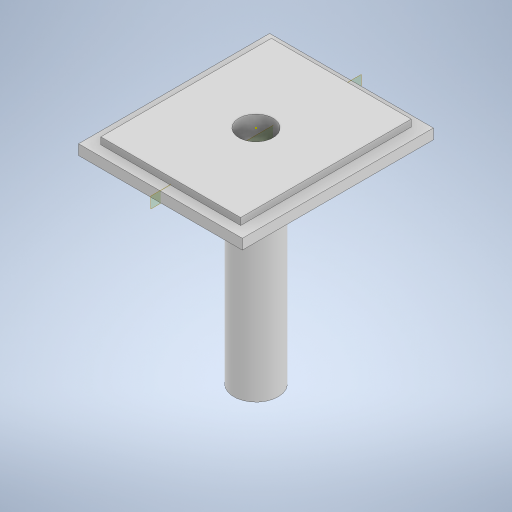
# Autodesk Inventor part: Tampa Eletroimã
Saved by Autodesk Inventor 2023 (Build 270158000, 158)
## iProperties
Created: 2023-03-07
Part Number: Tampa Eletroimã
Material: Genérico
Document SubType Name: Modeling
Designer: Inteli
Density: 1 g/cm^3
Appearance: Padrão
Author: Inteli
Autodesk Inventor part; units mm, degrees
ref_plane "YZ Plane" through (0, 0, 0) normal (1, 0, 0) x (0, 1, 0)
ref_plane "XZ Plane" through (0, 0, 0) normal (0, 1, 0) x (-1, 0, 0)
ref_plane "XY Plane" through (0, 0, 0) normal (0, 0, 1) x (1, 0, 0)
sketch "Esboço1" plane through (0, 0, 0) normal (0, 1, 0) x (-1, 0, 0)
  line L0 (24, 28) -> (-24, 28)
  line L1 (-24, 28) -> (-24, -28)
  line L2 (-24, -28) -> (24, -28)
  line L3 (24, -28) -> (24, 28)
  line L4 (24, 28) -> (-24, -28) construction
  line L5 (-24, 28) -> (24, -28) construction
  point P0 (0, 0)
  dimension "d0" = 48
  dimension "d1" = 56
  constraints: 12 end point, 2 midpoint, 2 parallel, 1 horizontal, 1 perpendicular
  measures "d0" distance of L2.end L1.end
  measures "d1" distance of L1.end L0.end
extrude "Base" add sketch "Esboço1" along normal blind 3
sketch "Esboço2" plane through (0, 3, 0) normal (0, 1, 0) x (1, 0, 0)
  line L0 (-20.5, -25) -> (20.5, -25)
  line L1 (20.5, -25) -> (20.5, 25)
  line L2 (20.5, 25) -> (-20.5, 25)
  line L3 (-20.5, 25) -> (-20.5, -25)
  line L4 (-20.5, -25) -> (20.5, 25) construction
  line L5 (20.5, -25) -> (-20.5, 25) construction
  line L6 (-24, 28) -> (-24, -28) projected
  point P0 (0, 0)
  dimension "d4" = 41
  dimension "d5" = 50
  constraints: 12 end point, 2 midpoint, 2 parallel, 1 horizontal, 1 perpendicular
  measures "d4" distance of L2.end L1.end
  measures "d5" distance of L1.end L0.end
extrude "Encaixe" add sketch "Esboço2" along normal blind 2
sketch "Esboço3" plane through (0, 0, 0) normal (0, -1, 0) x (1, 0, 0)
  circle A0 centre (0, 0) radius 6.5
  circle A1 centre (0, 0) radius 5
  dimension "d9" = 13
  dimension "d10" = 10
  constraints: 2 centre point, 2 coincident
  measures "d9" diameter of A0
  measures "d10" diameter of A1
extrude "Furo" cut sketch "Esboço3" against normal up to surface (5 mm away) contours A1
extrude "Haste" add sketch "Esboço3" along normal blind 60
ref_plane "Plano de trabalho2" through (0, 0, -28) normal (-1, 0, 0) x (0, 0, 1)
sketch "Esboço7" plane through (0, 0, -28) normal (-1, 0, 0) x (0, 0, 1)
  line L0 (21.5, 0) -> (16, 0)
  line L1 (34.5, 0) -> (21.5, 0) projected
  line L2 (23, -60) -> (23, 5) projected
  line L3 (28, -16.1877) -> (28, 0)
  line L4 (21.5, 0) -> (21.5, -60) projected
  arc A0 (21.5, -14.3209) -> (16, 0) centre (-14.0851, -19.7709) ccw
  line L5 (21.5, -14.3209) -> (21.5, 0)
  dimension "d31" = 36
  constraints: 6 end point, 2 collinear, 2 point on circle, 2 point on line, 1 centre point, 1 vertical
  measures "d31" radius of A0
revolve "Revolução2" add sketch "Esboço7" angle 360 about axis through (0, -16.1877, 0) along (0, 1, 0)
sketch "Esboço8" plane through (0, 5, 0) normal (0, 1, 0) x (1, 0, 0)
  point P0 (0, 0)
